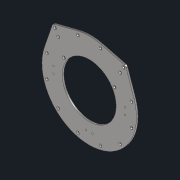
# Autodesk Inventor part: steel_plate6
Saved by Autodesk Inventor 2021 (Build 250183000, 183)
## iProperties
Created: 2021-07-12
Part Number: steel_plate6
Material: 鋼、炭素鋼
Document SubType Name: Sheet Metal
Designer: yuta0
Density: 7.85 g/cm^3
Sheet Metal Rule: Default_mm
Appearance: 半つや出し
購入先: カーボン
在庫数: 0.0
Author: yuta0
Autodesk Inventor part; units mm, degrees
ref_plane "YZ Plane" through (0, 0, 0) normal (1, 0, 0) x (0, 1, 0)
ref_plane "XZ Plane" through (0, 0, 0) normal (0, 1, 0) x (-1, 0, 0)
ref_plane "XY Plane" through (0, 0, 0) normal (0, 0, 1) x (1, 0, 0)
sketch "スケッチ1" plane through (0, 0, 0) normal (0, 0, 1) x (1, 0, 0)
  arc A0 (-63.8772, 21.8164) -> (63.8772, 21.8164) centre (0, 0) ccw
  line L0 (52.7853, 54.2928) -> (63.8772, 21.8164)
  line L1 (-94.5, 0) -> (94.5, 0) projected
  circle A1 centre (0, 53) radius 49 construction
  arc A2 (52.7853, 54.2928) -> (49.9924, 56.8749) centre (49, 53) ccw
  arc A3 (-49.9924, 56.8749) -> (-52.7853, 54.2928) centre (-49, 53) ccw
  circle A4 centre (0, 0) radius 67.5 construction
  line L2 (49.9924, 56.8749) -> (16.7471, 65.3895)
  line L3 (-63.8772, 21.8164) -> (-52.7853, 54.2928)
  line L4 (-49.9924, 56.8749) -> (-16.7471, 65.3895)
  arc A5 (16.7471, 65.3895) -> (-16.7471, 65.3895) centre (0, 0) ccw
  dimension "d0" = 135
  dimension "d63" = 98
  dimension "d64" = 53
  dimension "d65" = 8
  dimension "d66" = 8
  constraints: 13 point on circle, 8 end point, 8 tangent, 6 centre point, 2 coincident, 2 concentric, 2 horizontal alignment, 1 vertical alignment
  measures "d0" diameter of A0
  measures "d63" diameter of A1
  measures "d64" distance of point (0, 0) A1.centre
  measures "d65" diameter of A2
  measures "d66" diameter of A3
extrude "プレート1" add sketch "スケッチ1" along normal blind 2.3
sketch "スケッチ2" plane through (0, 0, 2.3) normal (0, 0, 1) x (1, 0, 0)
  circle A0 centre (0, 0) radius 38.5
  dimension "d2" = 77
  constraints: 1 centre point, 1 coincident
  measures "d2" diameter of A0
extrude "押し出し1" cut sketch "スケッチ2" against normal through all
sketch "スケッチ3" plane through (0, 0, 2.3) normal (0, 0, 1) x (1, 0, 0)
  circle A0 centre (0, 0) radius 62.5
  point P0 (16.1762, 60.3704)
  point P1 (-16.1762, 60.3704)
  point P2 (-44.1942, 44.1942)
  point P3 (-60.3704, 16.1762)
  point P4 (-60.3704, -16.1762)
  point P5 (-44.1942, -44.1942)
  point P6 (-16.1762, -60.3704)
  point P7 (16.1762, -60.3704)
  point P8 (44.1942, -44.1942)
  point P9 (60.3704, -16.1762)
  point P10 (60.3704, 16.1762)
  point P11 (44.1942, 44.1942)
  dimension "d5" = 125
  dimension "d8" = 360
  constraints: 1 coincident, 16 other
hole "穴1" at (16.1762, 60.3704, 2.3) at (-16.1762, 60.3704, 2.3) at (-44.1942, 44.1942, 2.3) at (-60.3704, 16.1762, 2.3) at (-60.3704, -16.1762, 2.3) at (-44.1942, -44.1942, 2.3) at (-16.1762, -60.3704, 2.3) at (16.1762, -60.3704, 2.3) at (44.1942, -44.1942, 2.3) at (60.3704, -16.1762, 2.3) at (60.3704, 16.1762, 2.3) at (44.1942, 44.1942, 2.3) direction (0, 0, -1) diameter 4.3 end through all clearance for "Flat Head Machine Screw" size "M4" standard "Ansi Metric M Profile"
sketch "スケッチ6" plane through (0, 0, 0) normal (0, 0, -1) x (-1, 0, 0)
  circle A0 centre (0, 0) radius 37.5
  line L0 (-4.75, -42.3) -> (4.75, -42.3)
  line L1 (-4.75, -37.5) -> (4.75, -37.5)
  circle A1 centre (0, -37.5) radius 4.8
  point P0 (-4.75, -51.1)
  point P1 (4.75, -51.1)
  dimension "d37" = 75
  dimension "d38" = 9.5
  dimension "d39" = 8.8
  dimension "d40" = 13.6
  dimension "d41" = 4.75
  constraints: 4 end point, 4 vertical alignment, 2 centre point, 2 horizontal, 2 tangent, 1 coincident, 1 horizontal alignment, 1 midpoint
  measures "d37" diameter of A0
  measures "d38" distance of point (-4.75, -51.1) point (4.75, -51.1)
  measures "d39" distance from line of point (4.75, -51.1) L0
  measures "d40" distance from line of point (4.75, -51.1) L1
  measures "d41" horizontal distance of L0.start point (0, 0)
hole "穴3" at (4.75, -51.1, 0) at (-4.75, -51.1, 0) direction (0, 0, 1) diameter 2.2 end through all clearance for "Socket Head Cap Screw" size "M2" standard "Ansi Metric M Profile"
sketch "スケッチ8" plane through (0, 0, 0) normal (0, 0, -1) x (-1, 0, 0)
  arc A0 (-49.9924, 56.8749) -> (-52.7853, 54.2928) centre (-49, 53) ccw projected
  arc A1 (52.7853, 54.2928) -> (49.9924, 56.8749) centre (49, 53) ccw projected
  point P0 (0, 0)
  point P1 (56.8749, 49.9924)
  point P2 (56.8749, -49.9924)
hole "穴4" at (-49, 53, 0) at (49, 53, 0) direction (0, 0, 1) diameter 4.5 depth 2.3 clearance for "Flat Head Machine Screw" size "M4" standard "Ansi Metric M Profile"
sketch "スケッチ9" plane through (0, 0, 0) normal (0, 0, -1) x (-1, 0, 0)
  circle A0 centre (0, 0) radius 42.5
  circle A1 centre (0, 53) radius 47.5
  point P0 (-36.2074, 22.2547)
  point P1 (36.2074, 22.2547)
  dimension "d74" = 85
  dimension "d75" = 95
  constraints: 4 point on circle, 2 centre point, 2 coincident
  measures "d74" diameter of A0
  measures "d75" diameter of A1
hole "穴5" at (-36.2074, 22.2547, 0) at (36.2074, 22.2547, 0) direction (0, 0, 1) diameter 4.5 depth 2.3 clearance for "Flat Head Machine Screw" size "M4" standard "Ansi Metric M Profile"
pattern_circular "円形状パターン2" count 4 over 360 about axis through (0, 0, -10) along (0, 0, 1) of "穴3" skipped copies 3
equation "\"d15\" = Thickness"
equation "\"d47\" = Thickness"
equation "\"d72\" = Thickness"
equation "\"d81\" = Thickness"
equation "\"d1\" = Thickness"
equation "\"BendRadius\" = Thickness"
equation "\"BendReliefWidth\" = Thickness"
equation "\"BendReliefDepth\" = 0.5 * Thickness"
equation "\"CornerReliefSize\" = 4 * Thickness"
equation "\"MinimumRemnant\" = 2 * Thickness"
equation "\"TransitionRadius\" = BendRadius"
equation "\"JacobiRadiusSize\" = BendRadius"
equation "\"GapSize\" = Thickness"
equation "\"Thickness\" = 2.3"
